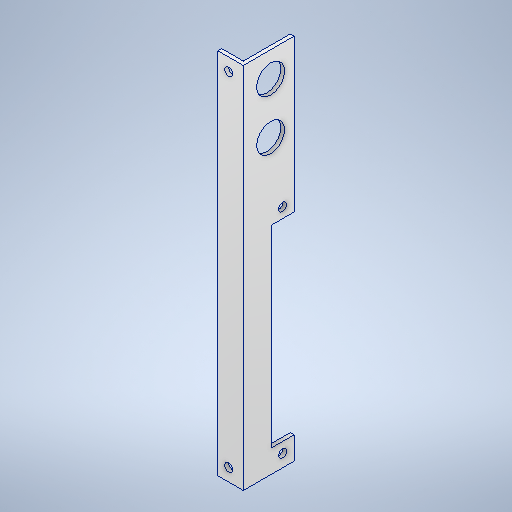
# Autodesk Inventor part: panel
Saved by Autodesk Inventor 2025 (Build 290162000, 162)
## iProperties
Created: 2024-04-25
Part Number: panel
Material: Hliník 6061
Document SubType Name: Modeling
Designer: rader
Density: 2.7 g/cm^3
Appearance: Hliník – plochý
Author: rader
Autodesk Inventor part; units mm, degrees
ref_plane "YZ Plane" through (0, 0, 0) normal (1, 0, 0) x (0, 1, 0)
ref_plane "XZ Plane" through (0, 0, 0) normal (0, 1, 0) x (-1, 0, 0)
ref_plane "XY Plane" through (0, 0, 0) normal (0, 0, 1) x (1, 0, 0)
sketch "Náčrt1" plane through (0, 0, 0) normal (0, 0, 1) x (1, 0, 0)
  line L0 (-10, 0) -> (0, 0)
  line L1 (0, 0) -> (0, 20)
  line L2 (0, 20) -> (-1.5, 20)
  line L3 (-1.5, 20) -> (-1.5, 1.5)
  line L4 (-1.5, 1.5) -> (-10, 1.5)
  line L5 (-10, 1.5) -> (-10, 0)
  line L6 (-12, 0) -> (2, 0) projected
  line L7 (0, 24) -> (0, -4) projected
  point P0 (0, 0)
  dimension "d0" = 20
  dimension "d1" = 10
  dimension "d2" = 1.5
  dimension "d3" = 1.5
  constraints: 12 end point, 5 perpendicular, 3 collinear, 1 horizontal
  measures "d0" distance of L0.end L1.end
  measures "d1" distance of L0.start L0.end
  measures "d2" distance between parallel lines of L3 L1
  measures "d3" distance between parallel lines of L4 L0
extrude "Vysunutí1" add sketch "Náčrt1" along normal mid plane 145
sketch "Náčrt2" plane through (-10, 1.5, 72.5) normal (0, 1, 0) x (1, 0, 0)
  line L0 (0, 0) -> (0, 145) projected
  line L1 (8.5, 0) -> (0, 0) projected
  line L2 (8.5, 145) -> (8.5, 0) projected
  line L3 (0, 145) -> (8.5, 145) projected
  point P0 (10, 72.5)
  point P1 (4.25, 140)
  point P2 (4.25, 5)
  point P3 (4.25, 0)
  dimension "d6" = 4.25
  dimension "d7" = 4.25
  dimension "d57" = 5
  dimension "d78" = 5
  constraints: 1 midpoint
  measures "d6" distance from line of L0 point (4.25, 5)
  measures "d7" distance from line of L0 point (4.25, 140)
  measures "d57" distance from line of point (4.25, 5) L1
  measures "d78" distance from line of L3 point (4.25, 140)
hole "Díra1" at (-5.75, 1.5, -67.5) at (-5.75, 1.5, 67.5) direction (0, -1, 0) diameter 3.2 end through all
sketch "Náčrt9" plane through (-1.5, 1.5, 72.5) normal (-1, 0, 0) x (0, 0, 1)
  line L0 (-145, 18.5) -> (0, 18.5) projected
  line L1 (0, 18.5) -> (0, 0) projected
  point P0 (-72.5, -1.5)
  point P1 (-10, 9.25)
  point P2 (-30, 9.25)
  dimension "d79" = 9.25
  dimension "d80" = 9.25
  dimension "d81" = 10
  dimension "d82" = 30
  measures "d79" distance from line of L0 point (-10, 9.25)
  measures "d80" distance from line of L0 point (-30, 9.25)
  measures "d81" distance from line of L1 point (-10, 9.25)
  measures "d82" distance from line of L1 point (-30, 9.25)
hole "Díra7" at (-1.5, 10.75, 62.5) at (-1.5, 10.75, 42.5) direction (1, 0, 0) diameter 11 end through all
sketch "Náčrt10" plane through (0, 0, 72.5) normal (1, 0, 0) x (0, 0, -1)
  circle A0 centre (30, 10.75) radius 5.5 projected
  circle A1 centre (10, 10.75) radius 5.5 projected
  line L0 (145, 20) -> (0, 20) projected
  line L1 (0, 0) -> (0, 20) projected
  line L2 (145, 0) -> (0, 0) projected
  line L3 (145, 20) -> (145, 0) projected
  line L4 (60, 20) -> (136, 20)
  line L5 (136, 20) -> (136, 11)
  line L6 (136, 11) -> (60, 11)
  line L7 (60, 11) -> (60, 20)
  point P0 (72.5, 0)
  point P1 (60, 15.5)
  dimension "d90" = 76
  dimension "d91" = 9
  dimension "d92" = 60
  constraints: 8 end point, 2 parallel, 1 horizontal, 1 midpoint, 1 perpendicular, 1 point on line
  measures "d90" distance of L5.end L6.end
  measures "d91" distance of L4.end L5.end
  measures "d92" distance from line of point (60, 15.5) L1
extrude "Vysunutí3" cut sketch "Náčrt10" against normal through all contours L5 L6 L7 L0
sketch "Náčrt11" plane through (0, 0, 72.5) normal (1, 0, 0) x (0, 0, -1)
  line L0 (136, 20) -> (136, 11) projected
  line L1 (136, 11) -> (60, 11) projected
  line L2 (60, 11) -> (60, 20) projected
  line L3 (60, 20) -> (0, 20) projected
  line L4 (0, 0) -> (0, 20) projected
  line L5 (145, 0) -> (0, 0) projected
  line L6 (145, 20) -> (145, 0) projected
  line L7 (145, 20) -> (136, 20) projected
  circle A0 centre (10, 10.75) radius 5.5 projected
  circle A1 centre (30, 10.75) radius 5.5 projected
  point P0 (72.5, 0)
  point P1 (56, 15.5)
  point P2 (140, 15.5)
  point P3 (140.5, 20)
  point P4 (136, 15.5)
  dimension "d96" = 4.5
  dimension "d97" = 4
  dimension "d98" = 4.5
  dimension "d99" = 4
  constraints: 2 midpoint
  measures "d96" vertical distance of point (140.5, 20) point (140, 15.5)
  measures "d97" distance of point (136, 15.5) point (140, 15.5)
  measures "d98" distance from line of L3 point (56, 15.5)
  measures "d99" distance from line of L2 point (56, 15.5)
hole "Díra8" at (0, 15.5, 16.5) at (0, 15.5, -67.5) direction (-1, 0, 0) diameter 3.2 end through all
